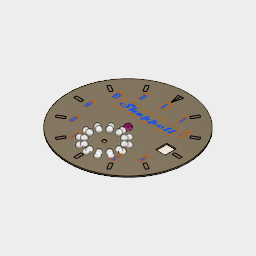
Dial (Autodesk Fusion 360 design; units mm, degrees)
Autodesk Fusion 360 part; units mm, degrees
sketch "Sketch1" plane through (0, 0, 0) normal (0, 1, 0) x (1, 0, 0)
  circle A0 centre (0, 0) radius 16.375
  dimension "d1" = 32.75
  measures "d1" diameter of A0
extrude "Extrude1" add sketch "Sketch1" along normal blind 0.35
sketch "Sketch3" plane through (0, 0.35, 0) normal (0, 1, 0) x (-1, 0, 0)
  circle A0 centre (0, 0) radius 16.375
  circle A1 centre (0, 0) radius 0.85
  line L0 (-9.1, 1.5) -> (-11.7, 1.5)
  line L1 (-11.7, 1.5) -> (-11.7, -1.5)
  line L2 (-11.7, -1.5) -> (-9.1, -1.5)
  line L3 (-9.1, -1.5) -> (-9.1, 1.5)
  circle A2 centre (0, 6.5) radius 0.5
  dimension "d4" = 1.7
  dimension "d5" = 2.6
  dimension "d6" = 3
  dimension "d7" = 1.5
  dimension "d8" = 9.1
  dimension "d9" = 1
  dimension "d10" = 6.5
  measures "d4" diameter of A1
  measures "d5" distance of L1.end L2.end
  measures "d6" distance of L0.end L1.end
  measures "d7" distance of A0.centre L2.end
  measures "d8" distance of A0.centre L3
  measures "d9" diameter of A2
  measures "d10" distance of A0.centre A2.centre
extrude "Extrude2" cut sketch "Sketch3" against normal through all contours A1 | L0 L1 L2 L3 | A2
sketch "Sketch4" plane through (0, 0.35, 0) normal (0, 1, 0) x (-1, 0, 0)
  line L0 (-9.1, -1.5) -> (-11.7, -1.5)
  line L1 (-11.7, -1.5) -> (-11.7, 1.5)
  line L2 (-11.7, 1.5) -> (-9.1, 1.5)
  line L3 (-9.1, 1.5) -> (-9.1, -1.5)
  circle A0 centre (0, 0) radius 0.85
  circle A1 centre (0, 6.5) radius 0.5
  circle A2 centre (0, 0) radius 16.375
  line L4 (0.375, 12.5) -> (-0.375, 12.5)
  line L5 (-0.375, 12.5) -> (-0.375, 14.5)
  line L6 (-0.375, 14.5) -> (0.375, 14.5)
  line L7 (0.375, 14.5) -> (0.375, 12.5)
  line L8 (-6.5748, 10.6378) -> (-7.5748, 12.3699)
  line L9 (-6.9252, 12.7449) -> (-5.9252, 11.0128)
  line L10 (-5.9252, 11.0128) -> (-6.5748, 10.6378)
  line L11 (-7.5748, 12.3699) -> (-6.9252, 12.7449)
  line L12 (-11.0128, 5.9252) -> (-12.7449, 6.9252)
  line L13 (-12.3699, 7.5748) -> (-10.6378, 6.5748)
  line L14 (-10.6378, 6.5748) -> (-11.0128, 5.9252)
  line L15 (-12.7449, 6.9252) -> (-12.3699, 7.5748)
  line L16 (-12.5, -0.375) -> (-14.5, -0.375)
  line L17 (-14.5, 0.375) -> (-12.5, 0.375)
  line L18 (-12.5, 0.375) -> (-12.5, -0.375)
  line L19 (-14.5, -0.375) -> (-14.5, 0.375)
  line L20 (-10.6378, -6.5748) -> (-12.3699, -7.5748)
  line L21 (-12.7449, -6.9252) -> (-11.0128, -5.9252)
  line L22 (-11.0128, -5.9252) -> (-10.6378, -6.5748)
  line L23 (-12.3699, -7.5748) -> (-12.7449, -6.9252)
  line L24 (-5.9252, -11.0128) -> (-6.9252, -12.7449)
  line L25 (-7.5748, -12.3699) -> (-6.5748, -10.6378)
  line L26 (-6.5748, -10.6378) -> (-5.9252, -11.0128)
  line L27 (-6.9252, -12.7449) -> (-7.5748, -12.3699)
  line L28 (6.5748, -10.6378) -> (7.5748, -12.3699)
  line L29 (6.9252, -12.7449) -> (5.9252, -11.0128)
  line L30 (5.9252, -11.0128) -> (6.5748, -10.6378)
  line L31 (7.5748, -12.3699) -> (6.9252, -12.7449)
  line L32 (11.0128, -5.9252) -> (12.7449, -6.9252)
  line L33 (12.3699, -7.5748) -> (10.6378, -6.5748)
  line L34 (10.6378, -6.5748) -> (11.0128, -5.9252)
  line L35 (12.7449, -6.9252) -> (12.3699, -7.5748)
  line L36 (12.5, 0.375) -> (14.5, 0.375)
  line L37 (14.5, -0.375) -> (12.5, -0.375)
  line L38 (12.5, -0.375) -> (12.5, 0.375)
  line L39 (14.5, 0.375) -> (14.5, -0.375)
  line L40 (10.6378, 6.5748) -> (12.3699, 7.5748)
  line L41 (12.7449, 6.9252) -> (11.0128, 5.9252)
  line L42 (11.0128, 5.9252) -> (10.6378, 6.5748)
  line L43 (12.3699, 7.5748) -> (12.7449, 6.9252)
  line L44 (5.9252, 11.0128) -> (6.9252, 12.7449)
  line L45 (7.5748, 12.3699) -> (6.5748, 10.6378)
  line L46 (6.5748, 10.6378) -> (5.9252, 11.0128)
  line L47 (6.9252, 12.7449) -> (7.5748, 12.3699)
  line L48 (0.75, -14.5) -> (-0.75, -14.5)
  line L49 (-0.75, -14.5) -> (0, -11.75)
  line L50 (0, -11.75) -> (0.75, -14.5)
  line L51 (0, -14.5) -> (0, -11.75)
  line L52 (-5, 6.5) -> (-4, 6.5)
  line L53 (-4.3301, 4) -> (-3.4641, 4.5)
  line L54 (-2.5, 2.1699) -> (-2, 3.0359)
  line L55 (0, 1.5) -> (0, 2.5)
  line L56 (2.5, 2.1699) -> (2, 3.0359)
  line L57 (4.3301, 4) -> (3.4641, 4.5)
  line L58 (5, 6.5) -> (4, 6.5)
  line L59 (4.3301, 9) -> (3.4641, 8.5)
  line L60 (2.5, 10.8301) -> (2, 9.9641)
  line L61 (0, 11.5) -> (0, 10.5)
  line L62 (-2.5, 10.8301) -> (-2, 9.9641)
  line L63 (-4.3301, 9) -> (-3.4641, 8.5)
  dimension "d12" = 0.75
  dimension "d13" = 2
  dimension "d14" = 14.5
  dimension "d15" = 0.375
  dimension "d17" = 360
  dimension "d18" = 2.75
  dimension "d19" = 1.5
  dimension "d20" = 14.5
  dimension "d21" = 0.75
  dimension "d24" = 5
  dimension "d25" = 1
  dimension "d27" = 360
  measures "d12" distance of L4.start L4.end
  measures "d13" distance of L4.start L6.end
  measures "d14" distance of A0.centre L6
  measures "d15" distance of A0.centre L4.start
  measures "d18" distance of L49.end L51.start
  measures "d19" distance of L48.start L48.end
  measures "d20" distance of A0.centre L48
  measures "d21" distance of A0.centre L48.end
  measures "d24" distance of A1.centre L52.start
  measures "d25" distance of L52.start L52.end
sketch "Sketch5" plane through (0, 0.35, 0) normal (0, 1, 0) x (-1, 0, 0)
  line L0 (6.985, -3.5778) -> (-7.6268, -3.5778) construction
  line L1 (-7.6268, -3.5778) -> (-7.6268, -6.5778) construction
  line L2 (-7.6268, -6.5778) -> (6.985, -6.5778) construction
  line L3 (6.985, -6.5778) -> (6.985, -3.5778) construction
  line L4 (0.4767, -9.049) -> (-0.7965, -9.049) construction
  line L5 (-0.7965, -9.049) -> (-0.7965, -11.549) construction
  line L6 (-0.7965, -11.549) -> (0.4767, -11.549) construction
  line L7 (0.4767, -11.549) -> (0.4767, -9.049) construction
  line L8 (-5.4546, -8.2) -> (-5.7, -8.2) construction
  line L9 (-5.7, -8.2) -> (-5.7, -10.7) construction
  line L10 (-5.7, -10.7) -> (-5.4546, -10.7) construction
  line L11 (-5.4546, -10.7) -> (-5.4546, -8.2) construction
  line L12 (-9.0419, -4.874) -> (-9.8, -4.874) construction
  line L13 (-9.8, -4.874) -> (-9.8, -7.374) construction
  line L14 (-9.8, -7.374) -> (-9.0419, -7.374) construction
  line L15 (-9.0419, -7.374) -> (-9.0419, -4.874) construction
  line L16 (-9.1553, 6.5) -> (-10, 6.5) construction
  line L17 (-10, 6.5) -> (-10, 4) construction
  line L18 (-10, 4) -> (-9.1553, 4) construction
  line L19 (-9.1553, 4) -> (-9.1553, 6.5) construction
  line L20 (-5.2603, 10) -> (-6, 10) construction
  line L21 (-6, 10) -> (-6, 7.5) construction
  line L22 (-6, 7.5) -> (-5.2603, 7.5) construction
  line L23 (-5.2603, 7.5) -> (-5.2603, 10) construction
  line L24 (5.6618, -8.1907) -> (4.9086, -8.1907) construction
  line L25 (4.9086, -8.1907) -> (4.9086, -10.6907) construction
  line L26 (4.9086, -10.6907) -> (5.6618, -10.6907) construction
  line L27 (5.6618, -10.6907) -> (5.6618, -8.1907) construction
  line L28 (5.7568, 10.0139) -> (5, 10.0139) construction
  line L29 (5, 10.0139) -> (5, 7.5139) construction
  line L30 (5, 7.5139) -> (5.7568, 7.5139) construction
  line L31 (5.7568, 7.5139) -> (5.7568, 10.0139) construction
  line L32 (9.7568, 6.5) -> (8.9817, 6.5) construction
  line L33 (8.9817, 6.5) -> (8.9817, 4) construction
  line L34 (8.9817, 4) -> (9.7568, 4) construction
  line L35 (9.7568, 4) -> (9.7568, 6.5) construction
  line L36 (11.2571, 0.9949) -> (10.5002, 0.9949) construction
  line L37 (10.5002, 0.9949) -> (10.5002, -1.5051) construction
  line L38 (10.5002, -1.5051) -> (11.2571, -1.5051) construction
  line L39 (11.2571, -1.5051) -> (11.2571, 0.9949) construction
  line L40 (9.7568, -4.9) -> (8.4141, -4.9) construction
  line L41 (8.4141, -4.9) -> (8.4141, -7.4) construction
  line L42 (8.4141, -7.4) -> (9.7568, -7.4) construction
  line L43 (9.7568, -7.4) -> (9.7568, -4.9) construction
